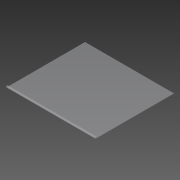
# Autodesk Inventor part: Part1
Saved by Autodesk Inventor 2013 (Build 170138000, 138)
## iProperties
Created: 2013-04-28
Part Number: Part1
Material: Polycarbonate, Clear
Document SubType Name: Sheet Metal
Designer: Chris
Density: 1.2 g/cm^3
Sheet Metal Rule: Default
Author: Chris
Autodesk Inventor part; units mm, degrees
ref_plane "YZ Plane" through (0, 0, 0) normal (1, 0, 0) x (0, 1, 0)
ref_plane "XZ Plane" through (0, 0, 0) normal (0, 1, 0) x (-1, 0, 0)
ref_plane "XY Plane" through (0, 0, 0) normal (0, 0, 1) x (1, 0, 0)
sketch "Sketch1" plane through (0, 0, 0) normal (0, 1, 0) x (-1, 0, 0)
  line L0 (0, 0) -> (1371.6, 0)
  line L1 (1371.6, 0) -> (1371.6, 1219.2)
  line L2 (1371.6, 1219.2) -> (0, 1219.2)
  line L3 (0, 1219.2) -> (0, 0)
  dimension "d0" = 1371.6
  dimension "d1" = 1219.2
  measures "d0" distance of L2.end L1.end
  measures "d1" distance of L1.end L0.end
extrude "Plate1" add sketch "Sketch1" along normal blind 5.3975
sketch "Sketch2" plane through (0, 0, 1213.8025) normal (0, 0, 1) x (1, 0, 0)
  line L0 (-1371.6, 0) -> (0, 0)
  line L1 (0, 0) -> (0, 25.4)
  line L2 (0, 25.4) -> (-1371.6, 25.4)
  line L3 (-1371.6, 25.4) -> (-1371.6, 0)
  constraints: 6 end point, 1 horizontal, 1 perpendicular, 1 vertical
edge flange "Flange1" height 25.4 angle 90 thickness 5.3975 bend radius 5.3975 thickness toward (0, 0, 1) relief tear relief width 5.3975 relief depth 2.6987 edges at (-685.8, 5.3975, 1219.2) wall of the first edge with corners at (-1371.6, 0, 1213.8025) (0, 0, 1213.8025) (0, 25.4, 1213.8025) (-1371.6, 25.4, 1213.8025)
bend "Bend1"
corner "Corner1"
sketch "Sketch3" plane through (0, 20.0025, 1219.2) normal (0, 1, 0) x (-1, 0, 0)
  line L0 (1371.6, 0) -> (0, 0)
  line L1 (0, 0) -> (0, -25.4)
  line L2 (0, -25.4) -> (1371.6, -25.4)
  line L3 (1371.6, -25.4) -> (1371.6, 0)
  constraints: 6 end point, 1 horizontal, 1 perpendicular, 1 vertical
edge flange "Flange2" height 25.4 angle 90 thickness 5.3975 bend radius 5.3975 thickness toward (0, 1, 0) relief tear relief width 5.3975 relief depth 2.6987 edges at (-685.8, 25.4, 1213.8025) wall of the first edge with corners at (-1371.6, 20.0025, 1219.2) (0, 20.0025, 1219.2) (0, 20.0025, 1193.8) (-1371.6, 20.0025, 1193.8)
bend "Bend2"
corner "Corner2"
equation "\"d3\" = BendReliefWidth"
equation "\"d4\" = BendReliefDepth"
equation "\"d5\" = MinimumRemnant"
equation "\"d6\" = BendRadius"
equation "\"d9\" = BendRadius"
equation "\"d10\" = CornerReliefSize"
equation "\"d11\" = GapSize"
equation "\"d12\" = JacobiRadiusSize"
equation "\"d13\" = BendReliefWidth"
equation "\"d14\" = BendReliefDepth"
equation "\"d15\" = MinimumRemnant"
equation "\"d16\" = BendRadius"
equation "\"d19\" = BendRadius"
equation "\"d20\" = CornerReliefSize"
equation "\"d21\" = GapSize"
equation "\"d22\" = JacobiRadiusSize"
equation "\"BendRadius\" = Thickness"
equation "\"BendReliefWidth\" = Thickness"
equation "\"BendReliefDepth\" = 0.5 * Thickness"
equation "\"CornerReliefSize\" = 4 * Thickness"
equation "\"MinimumRemnant\" = 2 * Thickness"
equation "\"TransitionRadius\" = BendRadius"
equation "\"JacobiRadiusSize\" = BendRadius"
equation "\"GapSize\" = Thickness"
equation "\"d2\" = BendRadius"
equation "\"Thickness\" = 5.3975"
body "Solid1"
